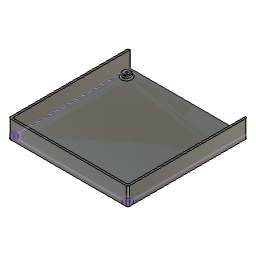
Bottom v3 (Autodesk Fusion 360 design; units mm, degrees)
Autodesk Fusion 360 part; units mm, degrees
note: some values were not read from the file. Set by a fixed rule: which sketch regions a step uses.
sketch "Base" plane through (0, 0, 0) normal (0, 0, 1) x (1, 0, 0)
  line L0 (2.5, 0) -> (177.5, 0)
  line L1 (180, 2.5) -> (180, 178)
  line L2 (177.5, 180.5) -> (2.5, 180.5)
  line L3 (0, 178) -> (0, 2.5)
  arc A0 (2.5, 180.5) -> (0, 178) centre (2.5, 178) ccw
  arc A1 (180, 178) -> (177.5, 180.5) centre (177.5, 178) ccw
  arc A2 (177.5, 0) -> (180, 2.5) centre (177.5, 2.5) ccw
  arc A3 (0, 2.5) -> (2.5, 0) centre (2.5, 2.5) ccw
  point P0 (180, 0)
  point P1 (0, 180.5)
  dimension "d1" = 180
  dimension "d2" = 180.5
  dimension "d3" = 2.5
  constraint horizontal L0
  constraint vertical L1
  constraint horizontal L2
  constraint vertical L3
  constraint coincident P1 L2
  constraint coincident P1 L3
  constraint tangent L2 A0
  constraint tangent L3 A0
  constraint tangent L1 A1
  constraint tangent L2 A1
  constraint equal A0 A1
  constraint coincident P0 L0
  constraint coincident P0 L1
  constraint tangent L0 A2
  constraint tangent L1 A2
  constraint equal A0 A2
  constraint coincident origin L0
  constraint coincident origin L3
  constraint tangent L0 A3
  constraint tangent L3 A3
  constraint equal A0 A3
  measures "d1" distance of origin P0
  measures "d2" distance of origin P1
  measures "d3" radius of A0
extrude "Extrude1" add sketch "Base" along normal blind 27
sketch "Cut Out Interior" plane through (0, 0, 27) normal (0, 0, 1) x (1, 0, 0)
  arc A0 (0, 2.5) -> (2.5, 0) centre (2.5, 2.5) ccw
  line L0 (2.5, 0) -> (177.5, 0)
  arc A1 (177.5, 0) -> (180, 2.5) centre (177.5, 2.5) ccw
  line L1 (180, 2.5) -> (180, 178)
  arc A2 (180, 178) -> (177.5, 180.5) centre (177.5, 178) ccw
  line L2 (177.5, 180.5) -> (2.5, 180.5)
  arc A3 (2.5, 180.5) -> (0, 178) centre (2.5, 178) ccw
  line L3 (0, 178) -> (0, 2.5)
  line L4 (3, 184.1293) -> (3, 5.5)
  line L5 (5.5, 3) -> (174.5, 3)
  line L6 (177, 5.5) -> (177, 184.1293)
  line L7 (174.5, 186.6293) -> (5.5, 186.6293)
  arc A4 (177, 184.1293) -> (174.5, 186.6293) centre (174.5, 184.1293) ccw
  arc A5 (174.5, 3) -> (177, 5.5) centre (174.5, 5.5) ccw
  arc A6 (3, 5.5) -> (5.5, 3) centre (5.5, 5.5) ccw
  arc A7 (5.5, 186.6293) -> (3, 184.1293) centre (5.5, 184.1293) ccw
  dimension "d44" = 2.5
  constraint parallel L3 L4
  constraint parallel L0 L5
  constraint parallel L1 L6
  constraint parallel L2 L7
  constraint tangent L6 A4
  constraint tangent L7 A4
  constraint tangent L5 A5
  constraint tangent L6 A5
  constraint equal A4 A5
  constraint tangent L4 A6
  constraint tangent L5 A6
  constraint equal A4 A6
  constraint tangent L4 A7
  constraint tangent L7 A7
  constraint equal A4 A7
  measures "d44" radius of A4
extrude "Extrude2" cut sketch "Cut Out Interior" against normal blind 24 contours L2 L4 L5 L6 A5 A6
sketch "Standoff 1" plane through (0, 0, 3) normal (0, 0, 1) x (-1, 0, 0)
  line L0 (-177, -180.5) -> (-3, -180.5)
  circle A0 centre (-168.83, -143.91) radius 6
  circle A1 centre (-168.83, -143.91) radius 1.75
  line L1 (-180, -2.5) -> (-180, -178)
  line L2 (-2.5, 0) -> (-177.5, 0)
  line L3 (-3, -180.5) -> (-3, -5.5)
  arc A2 (-3, -5.5) -> (-5.5, -3) centre (-5.5, -5.5) ccw
  line L4 (-5.5, -3) -> (-174.5, -3)
  arc A3 (-174.5, -3) -> (-177, -5.5) centre (-174.5, -5.5) ccw
  line L5 (-177, -5.5) -> (-177, -180.5)
  dimension "d17" = 12
  dimension "d18" = 36.59
  dimension "d20" = 3.5
  dimension "d29" = 11.17
  constraint concentric A0 A1
  measures "d17" diameter of A0
  measures "d18" distance of L0 A0.centre
  measures "d20" diameter of A1
  measures "d29" distance of A0.centre L1
extrude "Extrude3" add sketch "Standoff 1" along normal blind 6 contours A0
fillet "Fillet1" radius 1 1 edges at (174.424, 146.0797, 9)
fillet "Fillet2" radius 2 1 edges at (174.424, 141.7403, 3)
sketch "Sketch5" plane through (0, 0, 3) normal (0, 0, 1) x (-1, 0, 0)
  line L0 (-177, -180.5) -> (-3, -180.5)
  circle A0 centre (-168.83, -143.91) radius 8
  line L1 (-3, -180.5) -> (-3, -5.5)
  arc A1 (-3, -5.5) -> (-5.5, -3) centre (-5.5, -5.5) ccw
  line L2 (-5.5, -3) -> (-174.5, -3)
  arc A2 (-174.5, -3) -> (-177, -5.5) centre (-174.5, -5.5) ccw
  line L3 (-177, -5.5) -> (-177, -180.5)
sketch "Sketch6" plane through (0, 0, 3) normal (0, 0, 1) x (-1, 0, 0)
sketch "Standoff 2" plane through (0, 0, 3) normal (0, 0, 1) x (-1, 0, 0)
  circle A0 centre (-168.83, -11.83) radius 6
  circle A1 centre (-168.83, -11.83) radius 1.75
  line L0 (-2.5, 0) -> (-177.5, 0)
  line L1 (-180, -2.5) -> (-180, -178)
  point P0 (-168.83, -143.91)
  dimension "d32" = 12
  dimension "d33" = 3.5
  dimension "d35" = 11.17
  dimension "d45" = 132.08
  constraint concentric A0 A1
  measures "d32" diameter of A0
  measures "d33" diameter of A1
  measures "d35" distance of A0.centre L1
  measures "d45" distance of A0.centre P0
extrude "Extrude4" add sketch "Standoff 2" along normal blind 6
fillet "Fillet3" radius 1 1 edges at (174.424, 13.9997, 9)
fillet "Fillet4" radius 2 1 edges at (174.424, 9.6603, 3)
sketch "Sketch8" plane through (0, 0, 3) normal (0, 0, 1) x (-1, 0, 0)
  circle A0 centre (-10.75, -10.08) radius 6
  line L0 (-2.5, 0) -> (-177.5, 0)
  line L1 (0, -178) -> (0, -2.5)
  circle A1 centre (-10.75, -10.08) radius 1.75
  dimension "d46" = 12
  dimension "d47" = 10.08
  dimension "d48" = 10.75
  dimension "d49" = 3.5
  constraint concentric A0 A1
  measures "d46" diameter of A0
  measures "d47" distance of A0.centre L0
  measures "d48" distance of A0.centre L1
  measures "d49" diameter of A1
extrude "Extrude5" add sketch "Sketch8" along normal blind 6
fillet "Fillet5" radius 1 1 edges at (16.344, 12.2497, 9)
fillet "Fillet6" radius 2 1 edges at (16.344, 7.9103, 3)
sketch "Sketch9" plane through (0, 0, 3) normal (0, 0, 1) x (-1, 0, 0)
  circle A0 centre (-11.35, -166.78) radius 6
  line L0 (-3, -180.5) -> (-3, -5.5)
  line L1 (-177, -180.5) -> (-3, -180.5)
  circle A1 centre (-11.35, -166.78) radius 1.75
  dimension "d56" = 12
  dimension "d57" = 8.35
  dimension "d58" = 13.72
  dimension "d59" = 3.5
  constraint concentric A0 A1
  measures "d56" diameter of A0
  measures "d57" distance of A0.centre L0
  measures "d58" distance of A0.centre L1
  measures "d59" diameter of A1
extrude "Extrude6" add sketch "Sketch9" along normal blind 6
fillet "Fillet7" radius 1 1 edges at (16.944, 168.9497, 9)
fillet "Fillet8" radius 2 1 edges at (16.944, 164.6103, 3)
